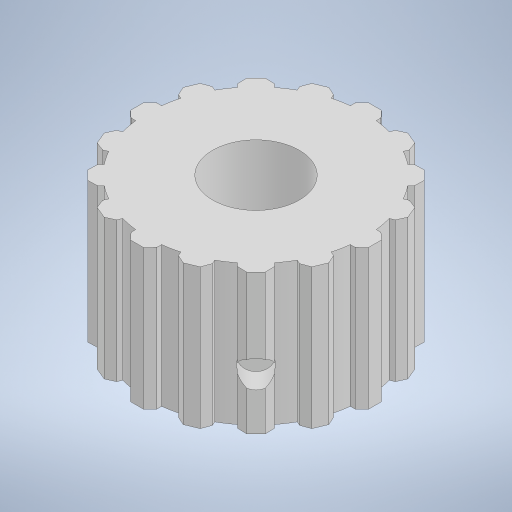
# Autodesk Inventor part: звезда_шестрерни
Saved by Autodesk Inventor 2023.1 (Build 271208000, 208)
## iProperties
Created: 2025-12-12
Part Number: звезда_шестрерни
Material: Типовые
Document SubType Name: Modeling
Designer: DELL
Density: 1 g/cm^3
Appearance: По умолчанию
Author: DELL
Autodesk Inventor part; units mm, degrees
ref_plane "YZ Plane" through (0, 0, 0) normal (1, 0, 0) x (0, 1, 0)
ref_plane "XZ Plane" through (0, 0, 0) normal (0, 1, 0) x (-1, 0, 0)
ref_plane "XY Plane" through (0, 0, 0) normal (0, 0, 1) x (1, 0, 0)
sketch "Эскиз1" plane through (0, 0, 0) normal (0, 1, 0) x (-1, 0, 0)
  line L0 (-11.25, -1.5) -> (-12.95, -1.5)
  line L1 (-13.75, -1.5) -> (-13.75, -0.75) construction
  line L2 (-13.75, 1.5) -> (-12.95, 1.5) construction
  line L3 (-11.25, 1.5) -> (-11.25, -1.5)
  circle A0 centre (0, 0) radius 12.5
  line L4 (-11.25, -1.5) -> (-13.75, 1.5) construction
  line L5 (-13.75, -1.5) -> (-11.25, 1.5) construction
  line L6 (-13.75, 0) -> (-11.25, 0) construction
  line L7 (-13.75, 0) -> (-13.75, 0.75)
  line L8 (-13.75, -0.75) -> (-12.95, -1.5)
  line L9 (-12.95, -1.5) -> (-12.95, 1.5) construction
  line L10 (-13.75, 0.75) -> (-12.95, 1.5)
  line L11 (-12.95, 1.5) -> (-11.25, 1.5)
  line L12 (-12.95, -1.5) -> (-13.75, -1.5) construction
  line L13 (-13.75, 0.75) -> (-13.75, 1.5) construction
  line L14 (-13.75, -0.75) -> (-13.75, 0)
  line L15 (-9.8196, -5.691) -> (-11.3902, -6.3416)
  line L16 (-12.1293, -6.6477) -> (-12.4163, -5.9548) construction
  line L17 (-13.2774, -3.8761) -> (-12.5383, -3.5699) construction
  line L18 (-10.9677, -2.9194) -> (-9.8196, -5.691)
  line L19 (-9.8196, -5.691) -> (-13.2774, -3.8761) construction
  line L20 (-12.1293, -6.6477) -> (-10.9677, -2.9194) construction
  line L21 (-12.7033, -5.2619) -> (-10.3936, -4.3052) construction
  line L22 (-12.7033, -5.2619) -> (-12.9904, -4.569)
  line L23 (-12.4163, -5.9548) -> (-11.3902, -6.3416)
  line L24 (-11.3902, -6.3416) -> (-12.5383, -3.5699) construction
  line L25 (-12.9904, -4.569) -> (-12.5383, -3.5699)
  line L26 (-12.5383, -3.5699) -> (-10.9677, -2.9194)
  line L27 (-11.3902, -6.3416) -> (-12.1293, -6.6477) construction
  line L28 (-12.9904, -4.569) -> (-13.2774, -3.8761) construction
  line L29 (-12.4163, -5.9548) -> (-12.7033, -5.2619)
  line L30 (-6.8943, -9.0156) -> (-8.0964, -10.2177)
  line L31 (-8.6621, -10.7834) -> (-9.1924, -10.253) construction
  line L32 (-10.7834, -8.6621) -> (-10.2177, -8.0964) construction
  line L33 (-9.0156, -6.8943) -> (-6.8943, -9.0156)
  line L34 (-6.8943, -9.0156) -> (-10.7834, -8.6621) construction
  line L35 (-8.6621, -10.7834) -> (-9.0156, -6.8943) construction
  line L36 (-9.7227, -9.7227) -> (-7.955, -7.955) construction
  line L37 (-9.7227, -9.7227) -> (-10.253, -9.1924)
  line L38 (-9.1924, -10.253) -> (-8.0964, -10.2177)
  line L39 (-8.0964, -10.2177) -> (-10.2177, -8.0964) construction
  line L40 (-10.253, -9.1924) -> (-10.2177, -8.0964)
  line L41 (-10.2177, -8.0964) -> (-9.0156, -6.8943)
  line L42 (-8.0964, -10.2177) -> (-8.6621, -10.7834) construction
  line L43 (-10.253, -9.1924) -> (-10.7834, -8.6621) construction
  line L44 (-9.1924, -10.253) -> (-9.7227, -9.7227)
  line L45 (-2.9194, -10.9677) -> (-3.5699, -12.5383)
  line L46 (-3.8761, -13.2774) -> (-4.569, -12.9904) construction
  line L47 (-6.6477, -12.1293) -> (-6.3416, -11.3902) construction
  line L48 (-5.691, -9.8196) -> (-2.9194, -10.9677)
  line L49 (-2.9194, -10.9677) -> (-6.6477, -12.1293) construction
  line L50 (-3.8761, -13.2774) -> (-5.691, -9.8196) construction
  line L51 (-5.2619, -12.7033) -> (-4.3052, -10.3936) construction
  line L52 (-5.2619, -12.7033) -> (-5.9548, -12.4163)
  line L53 (-4.569, -12.9904) -> (-3.5699, -12.5383)
  line L54 (-3.5699, -12.5383) -> (-6.3416, -11.3902) construction
  line L55 (-5.9548, -12.4163) -> (-6.3416, -11.3902)
  line L56 (-6.3416, -11.3902) -> (-5.691, -9.8196)
  line L57 (-3.5699, -12.5383) -> (-3.8761, -13.2774) construction
  line L58 (-5.9548, -12.4163) -> (-6.6477, -12.1293) construction
  line L59 (-4.569, -12.9904) -> (-5.2619, -12.7033)
  line L60 (1.5, -11.25) -> (1.5, -12.95)
  line L61 (1.5, -13.75) -> (0.75, -13.75) construction
  line L62 (-1.5, -13.75) -> (-1.5, -12.95) construction
  line L63 (-1.5, -11.25) -> (1.5, -11.25)
  line L64 (1.5, -11.25) -> (-1.5, -13.75) construction
  line L65 (1.5, -13.75) -> (-1.5, -11.25) construction
  line L66 (0, -13.75) -> (0, -11.25) construction
  line L67 (0, -13.75) -> (-0.75, -13.75)
  line L68 (0.75, -13.75) -> (1.5, -12.95)
  line L69 (1.5, -12.95) -> (-1.5, -12.95) construction
  line L70 (-0.75, -13.75) -> (-1.5, -12.95)
  line L71 (-1.5, -12.95) -> (-1.5, -11.25)
  line L72 (1.5, -12.95) -> (1.5, -13.75) construction
  line L73 (-0.75, -13.75) -> (-1.5, -13.75) construction
  line L74 (0.75, -13.75) -> (0, -13.75)
  line L75 (5.691, -9.8196) -> (6.3416, -11.3902)
  line L76 (6.6477, -12.1293) -> (5.9548, -12.4163) construction
  line L77 (3.8761, -13.2774) -> (3.5699, -12.5383) construction
  line L78 (2.9194, -10.9677) -> (5.691, -9.8196)
  line L79 (5.691, -9.8196) -> (3.8761, -13.2774) construction
  line L80 (6.6477, -12.1293) -> (2.9194, -10.9677) construction
  line L81 (5.2619, -12.7033) -> (4.3052, -10.3936) construction
  line L82 (5.2619, -12.7033) -> (4.569, -12.9904)
  line L83 (5.9548, -12.4163) -> (6.3416, -11.3902)
  line L84 (6.3416, -11.3902) -> (3.5699, -12.5383) construction
  line L85 (4.569, -12.9904) -> (3.5699, -12.5383)
  line L86 (3.5699, -12.5383) -> (2.9194, -10.9677)
  line L87 (6.3416, -11.3902) -> (6.6477, -12.1293) construction
  line L88 (4.569, -12.9904) -> (3.8761, -13.2774) construction
  line L89 (5.9548, -12.4163) -> (5.2619, -12.7033)
  line L90 (9.0156, -6.8943) -> (10.2177, -8.0964)
  line L91 (10.7834, -8.6621) -> (10.253, -9.1924) construction
  line L92 (8.6621, -10.7834) -> (8.0964, -10.2177) construction
  line L93 (6.8943, -9.0156) -> (9.0156, -6.8943)
  line L94 (9.0156, -6.8943) -> (8.6621, -10.7834) construction
  line L95 (10.7834, -8.6621) -> (6.8943, -9.0156) construction
  line L96 (9.7227, -9.7227) -> (7.955, -7.955) construction
  line L97 (9.7227, -9.7227) -> (9.1924, -10.253)
  line L98 (10.253, -9.1924) -> (10.2177, -8.0964)
  line L99 (10.2177, -8.0964) -> (8.0964, -10.2177) construction
  line L100 (9.1924, -10.253) -> (8.0964, -10.2177)
  line L101 (8.0964, -10.2177) -> (6.8943, -9.0156)
  line L102 (10.2177, -8.0964) -> (10.7834, -8.6621) construction
  line L103 (9.1924, -10.253) -> (8.6621, -10.7834) construction
  line L104 (10.253, -9.1924) -> (9.7227, -9.7227)
  line L105 (10.9677, -2.9194) -> (12.5383, -3.5699)
  line L106 (13.2774, -3.8761) -> (12.9904, -4.569) construction
  line L107 (12.1293, -6.6477) -> (11.3902, -6.3416) construction
  line L108 (9.8196, -5.691) -> (10.9677, -2.9194)
  line L109 (10.9677, -2.9194) -> (12.1293, -6.6477) construction
  line L110 (13.2774, -3.8761) -> (9.8196, -5.691) construction
  line L111 (12.7033, -5.2619) -> (10.3936, -4.3052) construction
  line L112 (12.7033, -5.2619) -> (12.4163, -5.9548)
  line L113 (12.9904, -4.569) -> (12.5383, -3.5699)
  line L114 (12.5383, -3.5699) -> (11.3902, -6.3416) construction
  line L115 (12.4163, -5.9548) -> (11.3902, -6.3416)
  line L116 (11.3902, -6.3416) -> (9.8196, -5.691)
  line L117 (12.5383, -3.5699) -> (13.2774, -3.8761) construction
  line L118 (12.4163, -5.9548) -> (12.1293, -6.6477) construction
  line L119 (12.9904, -4.569) -> (12.7033, -5.2619)
  line L120 (11.25, 1.5) -> (12.95, 1.5)
  line L121 (13.75, 1.5) -> (13.75, 0.75) construction
  line L122 (13.75, -1.5) -> (12.95, -1.5) construction
  line L123 (11.25, -1.5) -> (11.25, 1.5)
  line L124 (11.25, 1.5) -> (13.75, -1.5) construction
  line L125 (13.75, 1.5) -> (11.25, -1.5) construction
  line L126 (13.75, 0) -> (11.25, 0) construction
  line L127 (13.75, 0) -> (13.75, -0.75)
  line L128 (13.75, 0.75) -> (12.95, 1.5)
  line L129 (12.95, 1.5) -> (12.95, -1.5) construction
  line L130 (13.75, -0.75) -> (12.95, -1.5)
  line L131 (12.95, -1.5) -> (11.25, -1.5)
  line L132 (12.95, 1.5) -> (13.75, 1.5) construction
  line L133 (13.75, -0.75) -> (13.75, -1.5) construction
  line L134 (13.75, 0.75) -> (13.75, 0)
  line L135 (9.8196, 5.691) -> (11.3902, 6.3416)
  line L136 (12.1293, 6.6477) -> (12.4163, 5.9548) construction
  line L137 (13.2774, 3.8761) -> (12.5383, 3.5699) construction
  line L138 (10.9677, 2.9194) -> (9.8196, 5.691)
  line L139 (9.8196, 5.691) -> (13.2774, 3.8761) construction
  line L140 (12.1293, 6.6477) -> (10.9677, 2.9194) construction
  line L141 (12.7033, 5.2619) -> (10.3936, 4.3052) construction
  line L142 (12.7033, 5.2619) -> (12.9904, 4.569)
  line L143 (12.4163, 5.9548) -> (11.3902, 6.3416)
  line L144 (11.3902, 6.3416) -> (12.5383, 3.5699) construction
  line L145 (12.9904, 4.569) -> (12.5383, 3.5699)
  line L146 (12.5383, 3.5699) -> (10.9677, 2.9194)
  line L147 (11.3902, 6.3416) -> (12.1293, 6.6477) construction
  line L148 (12.9904, 4.569) -> (13.2774, 3.8761) construction
  line L149 (12.4163, 5.9548) -> (12.7033, 5.2619)
  line L150 (6.8943, 9.0156) -> (8.0964, 10.2177)
  line L151 (8.6621, 10.7834) -> (9.1924, 10.253) construction
  line L152 (10.7834, 8.6621) -> (10.2177, 8.0964) construction
  line L153 (9.0156, 6.8943) -> (6.8943, 9.0156)
  line L154 (6.8943, 9.0156) -> (10.7834, 8.6621) construction
  line L155 (8.6621, 10.7834) -> (9.0156, 6.8943) construction
  line L156 (9.7227, 9.7227) -> (7.955, 7.955) construction
  line L157 (9.7227, 9.7227) -> (10.253, 9.1924)
  line L158 (9.1924, 10.253) -> (8.0964, 10.2177)
  line L159 (8.0964, 10.2177) -> (10.2177, 8.0964) construction
  line L160 (10.253, 9.1924) -> (10.2177, 8.0964)
  line L161 (10.2177, 8.0964) -> (9.0156, 6.8943)
  line L162 (8.0964, 10.2177) -> (8.6621, 10.7834) construction
  line L163 (10.253, 9.1924) -> (10.7834, 8.6621) construction
  line L164 (9.1924, 10.253) -> (9.7227, 9.7227)
  line L165 (2.9194, 10.9677) -> (3.5699, 12.5383)
  line L166 (3.8761, 13.2774) -> (4.569, 12.9904) construction
  line L167 (6.6477, 12.1293) -> (6.3416, 11.3902) construction
  line L168 (5.691, 9.8196) -> (2.9194, 10.9677)
  line L169 (2.9194, 10.9677) -> (6.6477, 12.1293) construction
  line L170 (3.8761, 13.2774) -> (5.691, 9.8196) construction
  line L171 (5.2619, 12.7033) -> (4.3052, 10.3936) construction
  line L172 (5.2619, 12.7033) -> (5.9548, 12.4163)
  line L173 (4.569, 12.9904) -> (3.5699, 12.5383)
  line L174 (3.5699, 12.5383) -> (6.3416, 11.3902) construction
  line L175 (5.9548, 12.4163) -> (6.3416, 11.3902)
  line L176 (6.3416, 11.3902) -> (5.691, 9.8196)
  line L177 (3.5699, 12.5383) -> (3.8761, 13.2774) construction
  line L178 (5.9548, 12.4163) -> (6.6477, 12.1293) construction
  line L179 (4.569, 12.9904) -> (5.2619, 12.7033)
  line L180 (-1.5, 11.25) -> (-1.5, 12.95)
  line L181 (-1.5, 13.75) -> (-0.75, 13.75) construction
  line L182 (1.5, 13.75) -> (1.5, 12.95) construction
  line L183 (1.5, 11.25) -> (-1.5, 11.25)
  line L184 (-1.5, 11.25) -> (1.5, 13.75) construction
  line L185 (-1.5, 13.75) -> (1.5, 11.25) construction
  line L186 (0, 13.75) -> (0, 11.25) construction
  line L187 (0, 13.75) -> (0.75, 13.75)
  line L188 (-0.75, 13.75) -> (-1.5, 12.95)
  line L189 (-1.5, 12.95) -> (1.5, 12.95) construction
  line L190 (0.75, 13.75) -> (1.5, 12.95)
  line L191 (1.5, 12.95) -> (1.5, 11.25)
  line L192 (-1.5, 12.95) -> (-1.5, 13.75) construction
  line L193 (0.75, 13.75) -> (1.5, 13.75) construction
  line L194 (-0.75, 13.75) -> (0, 13.75)
  line L195 (-5.691, 9.8196) -> (-6.3416, 11.3902)
  line L196 (-6.6477, 12.1293) -> (-5.9548, 12.4163) construction
  line L197 (-3.8761, 13.2774) -> (-3.5699, 12.5383) construction
  line L198 (-2.9194, 10.9677) -> (-5.691, 9.8196)
  line L199 (-5.691, 9.8196) -> (-3.8761, 13.2774) construction
  line L200 (-6.6477, 12.1293) -> (-2.9194, 10.9677) construction
  line L201 (-5.2619, 12.7033) -> (-4.3052, 10.3936) construction
  line L202 (-5.2619, 12.7033) -> (-4.569, 12.9904)
  line L203 (-5.9548, 12.4163) -> (-6.3416, 11.3902)
  line L204 (-6.3416, 11.3902) -> (-3.5699, 12.5383) construction
  line L205 (-4.569, 12.9904) -> (-3.5699, 12.5383)
  line L206 (-3.5699, 12.5383) -> (-2.9194, 10.9677)
  line L207 (-6.3416, 11.3902) -> (-6.6477, 12.1293) construction
  line L208 (-4.569, 12.9904) -> (-3.8761, 13.2774) construction
  line L209 (-5.9548, 12.4163) -> (-5.2619, 12.7033)
  line L210 (-9.0156, 6.8943) -> (-10.2177, 8.0964)
  line L211 (-10.7834, 8.6621) -> (-10.253, 9.1924) construction
  line L212 (-8.6621, 10.7834) -> (-8.0964, 10.2177) construction
  line L213 (-6.8943, 9.0156) -> (-9.0156, 6.8943)
  line L214 (-9.0156, 6.8943) -> (-8.6621, 10.7834) construction
  line L215 (-10.7834, 8.6621) -> (-6.8943, 9.0156) construction
  line L216 (-9.7227, 9.7227) -> (-7.955, 7.955) construction
  line L217 (-9.7227, 9.7227) -> (-9.1924, 10.253)
  line L218 (-10.253, 9.1924) -> (-10.2177, 8.0964)
  line L219 (-10.2177, 8.0964) -> (-8.0964, 10.2177) construction
  line L220 (-9.1924, 10.253) -> (-8.0964, 10.2177)
  line L221 (-8.0964, 10.2177) -> (-6.8943, 9.0156)
  line L222 (-10.2177, 8.0964) -> (-10.7834, 8.6621) construction
  line L223 (-9.1924, 10.253) -> (-8.6621, 10.7834) construction
  line L224 (-10.253, 9.1924) -> (-9.7227, 9.7227)
  line L225 (-10.9677, 2.9194) -> (-12.5383, 3.5699)
  line L226 (-13.2774, 3.8761) -> (-12.9904, 4.569) construction
  line L227 (-12.1293, 6.6477) -> (-11.3902, 6.3416) construction
  line L228 (-9.8196, 5.691) -> (-10.9677, 2.9194)
  line L229 (-10.9677, 2.9194) -> (-12.1293, 6.6477) construction
  line L230 (-13.2774, 3.8761) -> (-9.8196, 5.691) construction
  line L231 (-12.7033, 5.2619) -> (-10.3936, 4.3052) construction
  line L232 (-12.7033, 5.2619) -> (-12.4163, 5.9548)
  line L233 (-12.9904, 4.569) -> (-12.5383, 3.5699)
  line L234 (-12.5383, 3.5699) -> (-11.3902, 6.3416) construction
  line L235 (-12.4163, 5.9548) -> (-11.3902, 6.3416)
  line L236 (-11.3902, 6.3416) -> (-9.8196, 5.691)
  line L237 (-12.5383, 3.5699) -> (-13.2774, 3.8761) construction
  line L238 (-12.4163, 5.9548) -> (-12.1293, 6.6477) construction
  line L239 (-12.9904, 4.569) -> (-12.7033, 5.2619)
  point P0 (-12.5, 0)
  point P1 (-11.5485, -4.7835)
  point P2 (-8.8388, -8.8388)
  point P3 (-4.7835, -11.5485)
  point P4 (0, -12.5)
  point P5 (4.7835, -11.5485)
  point P6 (8.8388, -8.8388)
  point P7 (11.5485, -4.7835)
  point P8 (12.5, 0)
  point P9 (11.5485, 4.7835)
  point P10 (8.8388, 8.8388)
  point P11 (4.7835, 11.5485)
  point P12 (0, 12.5)
  point P13 (-4.7835, 11.5485)
  point P14 (-8.8388, 8.8388)
  point P15 (-11.5485, 4.7835)
  point P16 (9.8356, -7.7143)
  point P17 (10.891, -6.1348)
  point P18 (12.0391, -3.3632)
  point P19 (12.4097, -1.5)
  point P20 (12.4097, 1.5)
  point P21 (12.0391, 3.3632)
  point P22 (10.891, 6.1348)
  point P23 (9.8356, 7.7143)
  point P24 (7.7143, 9.8356)
  point P25 (6.1348, 10.891)
  point P26 (3.3632, 12.0391)
  point P27 (1.5, 12.4097)
  point P28 (-1.5, 12.4097)
  point P29 (-3.3632, 12.0391)
  point P30 (-6.1348, 10.891)
  point P31 (-7.7143, 9.8356)
  point P32 (-9.8356, 7.7143)
  point P33 (-10.891, 6.1348)
  point P34 (-12.0391, 3.3632)
  point P35 (-12.4097, 1.5)
  point P36 (-12.4097, -1.5)
  point P37 (-12.0391, -3.3632)
  point P38 (-10.891, -6.1348)
  point P39 (-9.8356, -7.7143)
  point P40 (-7.7143, -9.8356)
  point P41 (-6.1348, -10.891)
  point P42 (-3.3632, -12.0391)
  point P43 (-1.5, -12.4097)
  point P44 (1.5, -12.4097)
  point P45 (3.3632, -12.0391)
  point P46 (6.1348, -10.891)
  point P47 (7.7143, -9.8356)
  dimension "d0" = 2.5
  dimension "d1" = 3
  dimension "d2" = 0.8
  dimension "d5" = 360
  constraints: 480 end point, 10 perpendicular, 8 parallel, 3 midpoint, 2 horizontal, 420 other
  measures "d0" distance of L2.start L3.start
  measures "d1" distance of L1.start L2.start
  measures "d2" distance of L1.start L0.end
extrude "Выдавливание1" add sketch "Эскиз1" along normal blind 16.2
sketch "Эскиз2" plane through (10.253, 0, 9.1924) normal (0.7071068, 0, 0.7071068) x (0.7071068, 0, -0.7071068)
  line L0 (-0.75, 0) -> (-0.75, 16.2) construction
  line L1 (-1.5, 16.2) -> (0, 16.2) construction
  circle A0 centre (-0.75, 6) radius 1.6
  line L2 (-1.5, 0) -> (0, 0) projected
  dimension "d9" = 3.2
  dimension "d10" = 6
  constraints: 2 end point, 1 centre point, 1 midpoint, 1 point on line
  measures "d9" diameter of A0
  measures "d10" distance from line of L2 A0.centre
extrude "Выдавливание2" cut sketch "Эскиз2" against normal blind 10
sketch "Эскиз3" plane through (0, 0, 0) normal (0, -1, 0) x (1, 0, 0)
  line L0 (0, 0) -> (12.7279, 12.7279) construction
  line L1 (0, 0) -> (18, 0) construction
  line L2 (-1.6502, 0) -> (16.3498, 0) construction
  line L3 (4.2139, 8.103) -> (8.103, 4.2139)
  line L4 (8.103, 4.2139) -> (9.8212, 5.9322)
  line L5 (9.8212, 5.9322) -> (5.9322, 9.8212)
  line L6 (5.9322, 9.8212) -> (4.2139, 8.103)
  line L7 (4.2139, 8.103) -> (9.8212, 5.9322) construction
  line L8 (8.103, 4.2139) -> (5.9322, 9.8212) construction
  point P0 (7.0176, 7.0176)
  dimension "d14" = 45
  dimension "d17" = 5.5
  dimension "d18" = 2.43
  constraints: 18 end point, 2 horizontal, 2 midpoint, 2 parallel, 2 point on line, 1 equal length, 1 perpendicular
  measures "d14" angle of L1 L0
  measures "d17" distance of L3.start L3.end
  measures "d18" distance of L4.end L3.end
extrude "Выдавливание3" cut sketch "Эскиз3" against normal blind 9
sketch "Эскиз4" plane through (0, 0, 0) normal (0, -1, 0) x (1, 0, 0)
  circle A0 centre (0, 0) radius 5
  dimension "d21" = 10
  constraints: 1 centre point, 1 coincident
  measures "d21" diameter of A0
extrude "Выдавливание4" cut sketch "Эскиз4" against normal blind 16.2
sketch "Эскиз5" plane through (-10.253, 0, -9.1924) normal (-0.7071068, 0, -0.7071068) x (-0.7071068, 0, 0.7071068)
  line L0 (-0.75, 0) -> (-0.75, 16.2) construction
  line L1 (-1.5, 16.2) -> (0, 16.2) construction
  circle A0 centre (-0.75, 5) radius 1.6
  line L2 (-1.5, 0) -> (0, 0) projected
  dimension "d24" = 3.2
  dimension "d25" = 5
  constraints: 2 end point, 1 centre point, 1 midpoint, 1 point on line
  measures "d24" diameter of A0
  measures "d25" distance from line of L2 A0.centre
extrude "Выдавливание5" cut sketch "Эскиз5" against normal blind 10
sketch "Эскиз6" plane through (0, 0, 0) normal (0, -1, 0) x (1, 0, 0)
  circle A0 centre (0, 0) radius 8 construction
  circle A1 centre (0, 8) radius 2
  circle A2 centre (0, 0) radius 8 construction
  circle A3 centre (-8, 0) radius 2
  circle A4 centre (0, 0) radius 8 construction
  circle A5 centre (0, -8) radius 2
  circle A6 centre (0, 0) radius 8 construction
  circle A7 centre (8, 0) radius 2
  dimension "d28" = 16
  dimension "d29" = 4
  dimension "d32" = 360
  constraints: 4 centre point, 3 coincident, 2 horizontal alignment, 2 vertical alignment, 23 other
  measures "d29" diameter of A1
extrude "Выдавливание6" cut sketch "Эскиз6" against normal blind 5
